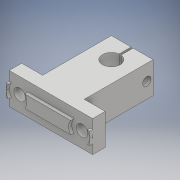
# Autodesk Inventor part: Suporte Eixos 8mm
Saved by Autodesk Inventor 2017 (Build 210142000, 142)
## iProperties
Created: 2020-08-02
Part Number: Suporte Eixos 8mm
Material: Generic
Document SubType Name: Modeling
Designer: ale
Density: 1 g/cm^3
Appearance: Default
Author: ale
Autodesk Inventor part; units mm, degrees
ref_plane "YZ Plane" through (0, 0, 0) normal (1, 0, 0) x (0, 1, 0)
ref_plane "XZ Plane" through (0, 0, 0) normal (0, 1, 0) x (-1, 0, 0)
ref_plane "XY Plane" through (0, 0, 0) normal (0, 0, 1) x (1, 0, 0)
sketch "Sketch1" plane through (0, 0, 0) normal (0, 0, 1) x (1, 0, 0)
  arc A0 (-0.4474, 4.2264) -> (0.4474, 4.2264) centre (0, 0) ccw
  line L0 (10, 10) -> (10, -23)
  line L1 (10, -23) -> (-10, -23)
  line L2 (-10, -23) -> (-10, 10)
  line L3 (-0.4474, 4.2264) -> (-0.4474, 10)
  line L4 (0.4474, 4.2264) -> (0.4474, 10)
  line L5 (-10, 10) -> (-0.4474, 10)
  line L6 (0.4474, 10) -> (10, 10)
  dimension "d2" = 8.5
  dimension "d3" = 20
  dimension "d7" = 23
  dimension "d43" = 10
  dimension "d44" = 10
  constraints: 14 end point, 2 point on circle, 1 centre point, 1 coincident, 1 parallel
  measures "d2" diameter of A0
  measures "d3" distance of L0.end L1.end
  measures "d7" distance from line of L1 point (0, 0)
  measures "d43" distance from line of L6 point (0, 0)
  measures "d44" distance from line of L5 point (0, 0)
extrude "Extrusion1" add sketch "Sketch1" along normal blind 15
sketch "Sketch2" plane through (-10, -23, 0) normal (0, -1, 0) x (1, 0, 0)
  line L0 (0, 0) -> (0, 15) projected
  line L1 (20, 0) -> (20, 15) projected
  line L2 (0, 0) -> (20, 15)
  line L3 (-10, 15) -> (30, 15)
  line L4 (30, 15) -> (30, 0)
  line L5 (30, 0) -> (-10, 0)
  line L6 (-10, 0) -> (-10, 15)
  line L7 (-10, 15) -> (30, 0) construction
  line L8 (30, 15) -> (-10, 0) construction
  point P0 (10, 0)
  point P1 (10, 7.5)
  dimension "d13" = 40
  dimension "d17" = 15
  constraints: 14 end point, 3 midpoint, 2 parallel, 1 horizontal, 1 perpendicular
  measures "d13" distance of L4.end L5.end
  measures "d17" distance between parallel lines of L5 L3
extrude "Extrusion2" add sketch "Sketch2" along normal blind 6
sketch "Sketch3" plane through (-10, -29, 0) normal (0, -1, 0) x (1, 0, 0)
  line L0 (-10, 10.5) -> (30, 10.5)
  line L1 (-10, 4.5) -> (30, 4.5)
  line L2 (-10, 4.5) -> (-10, 10.5)
  line L3 (-10, 0) -> (-10, 15) projected
  line L4 (30, 10.5) -> (30, 4.5)
  line L5 (30, 0) -> (30, 15) projected
  point P0 (10, 0)
  constraints: 8 end point, 2 collinear
extrude "Extrusion3" add sketch "Sketch3" along normal blind 1.5
sketch "Sketch4" plane through (-10, -30.5, 0) normal (0, -1, 0) x (1, 0, 0)
  line L0 (30, 4.5) -> (-10, 4.5) projected
  line L1 (-10, 10.5) -> (30, 10.5) projected
  line L2 (-10, 10.5) -> (-10, 4.5) projected
  line L3 (-10, 7.5) -> (-5, 7.5)
  line L4 (30, 15) -> (30, 0) projected
  line L5 (30, 7.5) -> (25, 7.5)
  point P0 (10, 0)
  dimension "d22" = 5
  dimension "d23" = 5
  constraints: 4 end point, 2 coincident, 2 horizontal, 2 midpoint
  measures "d22" distance of L3.start L3.end
  measures "d23" distance of L5.start L5.end
hole "Hole1" at (-15, -30.5, 7.5) at (15, -30.5, 7.5) direction (0, 1, 0) diameter 5.5 end through all counterbore diameter 10 counterbore depth 1.5
sketch "Sketch5" plane through (10, 10, 15) normal (1, 0, 0) x (0, 0, -1)
  line L0 (15, 0) -> (0, 0) projected
  line L1 (7.5, 0) -> (7.5, -3)
  point P0 (15, -10)
  dimension "d35" = 3
  constraints: 2 end point, 1 coincident, 1 midpoint, 1 vertical
  measures "d35" distance of L1.start L1.end
hole "Hole2" at (10, 7, 7.5) direction (-1, 0, 0) diameter 4 end through all
body "Solid1"
